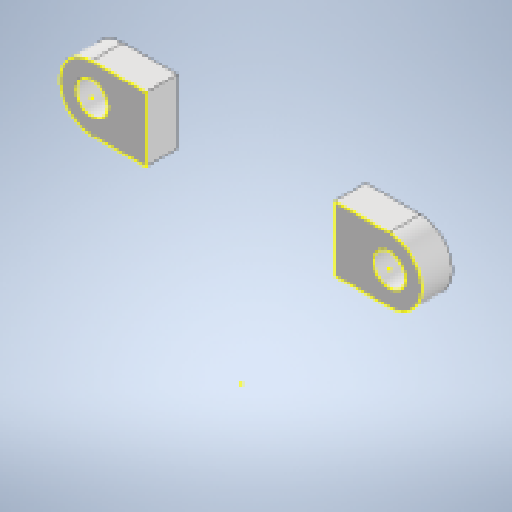
# Autodesk Inventor part: trzymacz
Saved by Autodesk Inventor 2023 (Build 270158000, 158)
## iProperties
Created: 2024-05-17
Part Number: trzymacz
Material: Ogólny
Document SubType Name: Modeling
Designer: kamil
Density: 1 g/cm^3
Appearance: Domyślna
Author: kamil
Autodesk Inventor part; units mm, degrees
ref_plane "YZ Plane" through (0, 0, 0) normal (1, 0, 0) x (0, 1, 0)
sketch "Szkic1" plane through (0, 0, 0) normal (0, 0, 1) x (1, 0, 0)
  circle A0 centre (-15.0668, 17.4281) radius 1.6 projected
  circle A1 centre (14.9332, 17.4281) radius 1.6 projected
  circle A2 centre (14.9332, 17.4281) radius 3.25
  circle A3 centre (-15.0668, 17.4281) radius 3.25
  line L0 (14.9332, 14.1781) -> (9.4332, 14.1781)
  line L1 (9.4332, 14.1781) -> (9.4332, 20.6781)
  line L2 (9.4332, 20.6781) -> (14.9332, 20.6781)
  line L3 (14.9332, 20.6781) -> (14.9332, 14.1781)
  line L4 (-15.0668, 14.1781) -> (-9.5668, 14.1781)
  line L5 (-9.5668, 14.1781) -> (-9.5668, 20.6781)
  line L6 (-9.5668, 20.6781) -> (-15.0668, 20.6781)
  line L7 (-15.0668, 20.6781) -> (-15.0668, 14.1781)
  point P0 (0, 0)
  dimension "d0" = 6.5
  dimension "d1" = 6.5
  dimension "d2" = 5.5
  dimension "d3" = 5.5
  constraints: 16 end point, 6 horizontal, 4 parallel, 2 coincident, 2 perpendicular, 6 other
  measures "d2" distance between parallel lines of L1 L3
  measures "d3" distance of L6.end L5.end
ref_plane "Płaszczyzna konstrukcyjna1" through (-7.6204, -2.8576, 3.15) normal (0, 0, 1) x (1, 0, 0)
extrude "Wyciągnięcie proste1" add sketch "Szkic1" along normal up to surface (3.15 mm away) contours A0 L7 A3 | A0 L7 A3 | L6 L5 L4 A3 | A1 L3 A2 | A1 L3 A2 | A2 L0 L1 L2
ref_plane "Płaszczyzna konstrukcyjna2" through (-10.5274, -25.5076, 4.15) normal (0, 0, -1) x (0, 1, 0)
sketch "Szkic4" plane through (9.4332, 20.6781, 3.15) normal (0, 0, 1) x (1, 0, 0)
  line L0 (0.5964, -6.1857) -> (-19.4036, -6.1857) projected
  line L1 (-19.4036, -6.1857) -> (-19.4036, -46.1857) projected
  line L2 (0.5964, -46.1857) -> (-19.4036, -46.1857) projected
  line L3 (0.5964, -6.1857) -> (0.5964, -46.1857) projected
  line L4 (-21.4036, -26.1857) -> (2.5964, -26.1857)
  line L5 (2.5964, -26.1857) -> (2.5964, -21.1857)
  line L6 (2.5964, -21.1857) -> (-21.4036, -21.1857)
  line L7 (-21.4036, -21.1857) -> (-21.4036, -26.1857)
  circle A0 centre (-24.5, -3.25) radius 1.6 projected
  line L8 (-19, -6.5) -> (-24.5, -6.5) projected
  line L9 (-19, 0) -> (-19, -6.5) projected
  line L10 (-24.5, 0) -> (-19, 0) projected
  arc A1 (-24.5, 0) -> (-24.5, -6.5) centre (-24.5, -3.25) ccw projected
  arc A2 (5.5, -6.5) -> (5.5, 0) centre (5.5, -3.25) ccw projected
  line L11 (0, 0) -> (5.5, 0) projected
  line L12 (0, -6.5) -> (0, 0) projected
  line L13 (5.5, -6.5) -> (0, -6.5) projected
  circle A3 centre (5.5, -3.25) radius 1.6 projected
  line L14 (-19, 0) -> (0, 0)
  point P0 (-9.4332, -20.6781)
  point P1 (-9.4036, -26.1857)
  point P2 (-9.4036, -46.1857)
  point P3 (0.5964, -21.1857)
  point P4 (0.5964, -6.5)
  point P5 (-19.4036, -6.5)
  point P6 (-19.4036, -21.1857)
  dimension "d15" = 5
  dimension "d16" = 15
  dimension "d17" = 2
  constraints: 10 end point, 2 horizontal, 2 midpoint, 2 parallel, 1 perpendicular, 1 vertical alignment
  measures "d15" distance of L5.end L4.end
  measures "d16" distance between parallel lines of L0 L6
  measures "d17" distance between parallel lines of L1 L7
extrude "Wyciągnięcie proste4" add sketch "Szkic4" along normal blind 1 contours L3 L13 L12 L0 | L0 L12 L11 A2 L13 L3 | L12 L13 L3 L6 L1 L8 L9 L0 | L0 L9 L14 L12 | L9 L8 L1 L0 | L0 L1 L8 A1 L10 L9 | L6 L5 L4 L3 | L3 L4 L1 L6 | L1 L4 L7 L6
sketch "Szkic5" plane through (9.4332, 20.6781, 4.15) normal (0, 0, 1) x (1, 0, 0)
  line L0 (-21.4036, -21.1857) -> (-21.4036, -26.1857) projected
  line L1 (2.5964, -21.1857) -> (0.5964, -21.1857) projected
  line L2 (0.5964, -21.1857) -> (0.5964, -6.5) projected
  line L3 (0.5964, -6.5) -> (5.5, -6.5) projected
  arc A0 (5.5, -6.5) -> (5.5, 0) centre (5.5, -3.25) ccw projected
  line L4 (5.5, 0) -> (-24.5, 0) projected
  arc A1 (-24.5, 0) -> (-24.5, -6.5) centre (-24.5, -3.25) ccw projected
  line L5 (-24.5, -6.5) -> (-19.4036, -6.5) projected
  line L6 (-19.4036, -6.5) -> (-19.4036, -21.1857) projected
  line L7 (-19.4036, -21.1857) -> (-21.4036, -21.1857) projected
  line L8 (-21.4036, -21.1857) -> (-21.4036, -26.1857) projected
  line L9 (-21.4036, -26.1857) -> (2.5964, -26.1857) projected
  line L10 (2.5964, -26.1857) -> (2.5964, -21.1857) projected
  circle A2 centre (5.5, -3.25) radius 1.6 projected
  circle A3 centre (-24.5, -3.25) radius 1.6 projected
  line L11 (-21.4036, -26.1857) -> (-19.6036, -26.1857)
  line L12 (-19.6036, -26.1857) -> (-19.6036, -21.1857)
  line L13 (-19.6036, -21.1857) -> (-21.4036, -21.1857)
  line L14 (-21.4036, -21.1857) -> (-21.4036, -26.1857)
  line L15 (2.5964, -26.1857) -> (2.5964, -21.1857) projected
  line L16 (2.5964, -26.1857) -> (0.7964, -26.1857)
  line L17 (0.7964, -26.1857) -> (0.7964, -21.1857)
  line L18 (0.7964, -21.1857) -> (2.5964, -21.1857)
  line L19 (2.5964, -21.1857) -> (2.5964, -26.1857)
  point P0 (-9.4332, -20.6781)
  point P1 (0.7964, -26.1857)
  dimension "d20" = 1.8
  dimension "d21" = 1.8
  constraints: 16 end point, 4 parallel, 2 horizontal, 2 perpendicular, 2 point on line
  measures "d20" distance of L13.end L12.end
  measures "d21" distance of L17.end L18.end
extrude "Wyciągnięcie proste5" add sketch "Szkic5" along normal blind 9.5 contours L7 L12 L9 L0 | L17 L1 L10 L9
sketch "Szkic6" plane through (9.4332, 20.6781, 13.65) normal (0, 0, 1) x (1, 0, 0)
  line L0 (-19.6036, -21.1857) -> (-21.4036, -21.1857) projected
  line L1 (-21.4036, -21.1857) -> (-21.4036, -26.1857) projected
  line L2 (-21.4036, -26.1857) -> (-19.6036, -26.1857) projected
  line L3 (-19.6036, -26.1857) -> (-19.6036, -21.1857) projected
  line L4 (0.7964, -26.1857) -> (2.5964, -26.1857) projected
  line L5 (2.5964, -26.1857) -> (2.5964, -21.1857) projected
  line L6 (2.5964, -21.1857) -> (0.7964, -21.1857) projected
  line L7 (0.7964, -21.1857) -> (0.7964, -26.1857) projected
  line L8 (-21.4036, -21.1857) -> (-21.4036, -26.1857) projected
  line L9 (-21.4036, -26.1857) -> (2.5964, -26.1857)
  line L10 (2.5964, -26.1857) -> (2.5964, -21.1857)
  line L11 (2.5964, -21.1857) -> (-21.4036, -21.1857)
  line L12 (-21.4036, -21.1857) -> (-21.4036, -26.1857)
  point P0 (-9.4332, -20.6781)
  constraints: 8 end point, 2 parallel, 1 horizontal, 1 perpendicular
extrude "Wyciągnięcie proste6" add sketch "Szkic6" along normal blind 2
fillet "Zaokrąglenie3" radius 1 4 edges at (12.0296, -3.0076, 15.65) (-11.9704, -3.0076, 15.65) (12.0296, -3.0076, 3.15) (-11.9704, -3.0076, 3.15)
sketch "Szkic7" plane through (9.4332, 20.6781, 4.15) normal (0, 0, 1) x (1, 0, 0)
  line L0 (0.7964, -26.1857) -> (0.7964, -21.1857) projected
  line L1 (0.7964, -21.1857) -> (0.5964, -21.1857) projected
  line L2 (0.5964, -21.1857) -> (0.5964, -6.5) projected
  line L3 (0.5964, -6.5) -> (5.5, -6.5) projected
  arc A0 (5.5, -6.5) -> (5.5, 0) centre (5.5, -3.25) ccw projected
  line L4 (5.5, 0) -> (-24.5, 0) projected
  arc A1 (-24.5, 0) -> (-24.5, -6.5) centre (-24.5, -3.25) ccw projected
  line L5 (-24.5, -6.5) -> (-19.4036, -6.5) projected
  line L6 (-19.4036, -6.5) -> (-19.4036, -21.1857) projected
  line L7 (-19.4036, -21.1857) -> (-19.6036, -21.1857) projected
  line L8 (-19.6036, -21.1857) -> (-19.6036, -26.1857) projected
  line L9 (-19.6036, -26.1857) -> (0.7964, -26.1857) projected
  circle A2 centre (5.5, -3.25) radius 1.6 projected
  circle A3 centre (-24.5, -3.25) radius 1.6 projected
  line L10 (-19.4036, -6.5) -> (0.5964, -6.5)
  line L11 (-19, -6.5) -> (-19, 0) projected
  point P0 (-9.4332, -20.6781)
  constraints: 2 end point, 1 perpendicular
extrude "Wyciągnięcie proste7" add sketch "Szkic7" along normal blind 2 contours L10 L11 L4 A0 L3 | L10 L5 A1 L4 L11
sketch "Szkic8" plane through (9.4332, 20.6781, 6.15) normal (0, 0, 1) x (1, 0, 0)
  circle A0 centre (5.5, -3.25) radius 1.6 projected
  circle A1 centre (-24.5, -3.25) radius 1.6 projected
  circle A2 centre (5.5, -3.25) radius 2.85
  circle A3 centre (-24.5, -3.25) radius 2.85
  line L0 (8.35, -4.8954) -> (5.5, -6.5409)
  line L1 (5.5, -6.5409) -> (2.65, -4.8954)
  line L2 (2.65, -4.8954) -> (2.65, -1.6046)
  line L3 (2.65, -1.6046) -> (5.5, 0.0409)
  line L4 (5.5, 0.0409) -> (8.35, -1.6046)
  line L5 (8.35, -1.6046) -> (8.35, -4.8954)
  line L6 (5.5, 0) -> (-24.5, 0) projected
  arc A4 (-24.5, 0) -> (-24.5, -6.5) centre (-24.5, -3.25) ccw projected
  line L7 (-24.5, -6.5) -> (5.5, -6.5) projected
  arc A5 (5.5, -6.5) -> (5.5, 0) centre (5.5, -3.25) ccw projected
  circle A6 centre (-24.5, -3.25) radius 1.6 projected
  circle A7 centre (5.5, -3.25) radius 1.6 projected
  line L8 (-27.35, -1.6046) -> (-24.5, 0.0409)
  line L9 (-24.5, 0.0409) -> (-21.65, -1.6046)
  line L10 (-21.65, -1.6046) -> (-21.65, -4.8954)
  line L11 (-21.65, -4.8954) -> (-24.5, -6.5409)
  line L12 (-24.5, -6.5409) -> (-27.35, -4.8954)
  line L13 (-27.35, -4.8954) -> (-27.35, -1.6046)
  point P0 (-9.4332, -20.6781)
  point P1 (8.35, -3.25)
  point P2 (-27.35, -3.25)
  point P3 (-24.5722, -0.0008)
  point P4 (-27.2778, -1.5629)
  point P5 (-27.35, -1.688)
  point P6 (-27.35, -4.812)
  point P7 (-27.2778, -4.9371)
  point P8 (-24.5722, -6.4992)
  point P9 (5.5722, -6.4992)
  point P10 (8.2778, -4.9371)
  point P11 (8.35, -4.812)
  point P12 (8.35, -1.688)
  point P13 (8.2778, -1.5629)
  point P14 (5.5722, -0.0008)
  dimension "d29" = 5.7
  dimension "d30" = 5.7
  constraints: 24 end point, 4 coincident, 2 horizontal alignment, 2 midpoint, 30 other
extrude "Wyciągnięcie proste8" cut sketch "Szkic8" against normal blind 2 contours A0 | A1 | A2 | L5 A5 L0 A2 | A2 L4 A5 L5 | L5 A5 | A2 L3 L6 A5 L4 | L4 A5 | L0 A5 L7 L1 A2 | L0 A5 | A5 L4 L5 | L5 L0 A5 | A2 L2 L3 | A5 L6 L3 L4 | L1 L2 A2 | L0 L1 L7 A5 | L9 A3 L8 A4 L6 | L6 A4 L8 L9 | L11 L12 A4 L7 | L7 A4 L12 A3 L11 | L9 L10 A3 | A3 | A3 L10 L11 | L8 A4 | A3 L13 A4 L8 | A4 L12 | L12 A4 L13 A3 | A4 L13 L8 | L13 A4 | L12 L13 A4
sketch "Szkic10" plane through (0, 0, 0) normal (0, 0, -1) x (-1, 0, 0)
  line L0 (9.5668, 14.1781) -> (9.5668, 20.6781) projected
  line L1 (15.0668, 14.1781) -> (9.5668, 14.1781) projected
  arc A0 (15.0668, 14.1781) -> (15.0668, 20.6781) centre (15.0668, 17.4281) ccw projected
  line L2 (9.5668, 20.6781) -> (15.0668, 20.6781) projected
  circle A1 centre (15.0668, 17.4281) radius 1.6 projected
  line L3 (-14.9332, 20.6781) -> (-9.4332, 20.6781) projected
  arc A2 (-14.9332, 20.6781) -> (-14.9332, 14.1781) centre (-14.9332, 17.4281) ccw projected
  line L4 (-9.4332, 14.1781) -> (-14.9332, 14.1781) projected
  line L5 (-9.4332, 20.6781) -> (-9.4332, 14.1781) projected
  circle A3 centre (-14.9332, 17.4281) radius 1.6 projected
  point P0 (0, 0)
extrude "Wyciągnięcie proste9" cut sketch "Szkic10" against normal up to surface (3.15 mm away)
fillet "Zaokrąglenie4" radius 2 2 edges at (-9.9704, 14.1781, 3.65) (10.0296, 14.1781, 3.65)
fillet "Zaokrąglenie5" radius 0.2 2 edges at (-9.9704, -0.5076, 3.65) (10.0296, -0.5076, 3.65)
